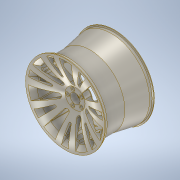
# Autodesk Inventor part: RIM
Saved by Autodesk Inventor 2020.2 (Build 242310000, 310)
## iProperties
RuleStatus: InUse
AfterAnyParamChange0: DARule
Created: 2019-05-23
Part Number: RIM
Material: Titanium
Document SubType Name: Modeling
Designer: Autodesk Developer Network
Density: 4.51 g/cm^3
Appearance: Titanium
Mass: 15996.9 g
Surface Area: 6136.53 cm^2
Volume: 3546.98 cm^3
Author: Autodesk Developer Network
Autodesk Inventor part; units mm, degrees
ref_plane "YZ Plane" through (0, 0, 0) normal (1, 0, 0) x (0, 1, 0)
ref_plane "XZ Plane" through (0, 0, 0) normal (0, 1, 0) x (-1, 0, 0)
sketch "Sketch1" plane through (0, 0, 0) normal (1, 0, 0) x (0, 1, 0)
  line L0 (203.2, 50.8) -> (203.2, 47.625)
  line L1 (203.2, 47.625) -> (196.85, 45.3138)
  line L2 (196.85, 45.3138) -> (196.85, 32.6138)
  line L3 (196.85, 32.6138) -> (177.8, 19.2748)
  line L4 (177.8, 19.2748) -> (177.8, -76.9759)
  line L5 (177.8, -76.9759) -> (196.85, -185.0138)
  line L6 (196.85, -185.0138) -> (196.85, -197.7138)
  line L7 (196.85, -197.7138) -> (203.2, -200.025)
  line L8 (203.2, -200.025) -> (203.2, -203.2)
  line L9 (203.2, -203.2) -> (190.5, -198.5776)
  line L10 (190.5, -198.5776) -> (190.5, -185.8776)
  line L11 (190.5, -185.8776) -> (158.75, -67.385)
  line L12 (158.75, -67.385) -> (158.75, 20.9537)
  line L13 (158.75, 20.9537) -> (165.1, 25.4)
  line L14 (165.1, 25.4) -> (154.94, 35.56)
  arc A0 (203.2, 50.8) -> (50.8, 0) centre (244.775, -327.9249) ccw
  arc A1 (154.94, 35.56) -> (50.8, -38.1) centre (319.7795, -307.9352) ccw
  line L15 (50.8, -38.1) -> (0, -38.1)
  line L16 (50.8, 0) -> (0, 0)
  line L17 (0, 0) -> (0, -38.1)
  dimension "w" = 254
  dimension "RimDia" = 203.2
  dimension "d2" = 381
  dimension "d3" = 381
  dimension "d5" = 6.35
  dimension "d6" = 110
  dimension "d7" = 3.175
  dimension "d8" = 3.175
  dimension "d9" = 110
  dimension "d10" = 19.05
  dimension "d11" = 125
  dimension "d14" = 12.7
  dimension "d15" = 50.8
  dimension "d16" = 38.1
  dimension "Width_angle2" = 170
  dimension "d18" = 12.7
  dimension "d19" = 6.35
  dimension "d20" = 19.05
  dimension "Width_angle1" = 165
  dimension "d22" = 125
  dimension "d24" = 50.8
  dimension "d25" = 50.8
  dimension "d28" = 38.1
  dimension "d29" = 25.4
  dimension "d30" = 48.26
  dimension "d31" = 15.24
  dimension "d32" = 18.1862
  constraints: 36 end point, 6 point on line, 5 parallel, 4 point on circle, 2 centre point, 2 horizontal, 1 perpendicular, 1 vertical
  measures "w" distance of L8.end L0.start
  measures "RimDia" horizontal distance of point (0, 0) L0.start
  measures "d2" radius of A0
  measures "d3" radius of A1
  measures "d5" distance between parallel lines of L0 L2
  measures "d6" angle of L2 L1
  measures "d7" distance of L0.start L0.end
  measures "d8" distance of L7.end L8.end
  measures "d9" angle of L6 L7
  measures "d10" distance between parallel lines of L4 L2
  measures "d11" angle of L4 L3
  measures "d14" distance of L1.end L2.end
  measures "d15" vertical distance of point (0, 0) L0.start
  measures "d16" distance of L16.end L15.end
  measures "Width_angle2" angle of L4 L5
  measures "d18" distance of L9.end L10.end
  measures "d19" distance between parallel lines of L10 L6
  measures "d20" distance between parallel lines of L12 L4
  measures "Width_angle1" angle of L11 L12
  measures "d22" angle of L12 L13
  measures "d24" distance of L15.start L15.end
  measures "d25" distance of L16.start L16.end
  measures "d28" horizontal distance of L0.start L13.end
  measures "d29" vertical distance of L13.end L0.start
  measures "d30" horizontal distance of L14.end L0.start
  measures "d31" vertical distance of L14.end L0.start
  measures "d32" vertical distance of L5.end L8.end
revolve "Revolution1" add sketch "Sketch1" angle 360 about axis through (0, 0, 0) along (0, 0, -1)
ref_plane "Work Plane1" through (0, 0, 127) normal (0, 0, 1) x (1, 0, 0)
sketch "Sketch2" plane through (0, 0, 127) normal (0, 0, 1) x (1, 0, 0)
  line L0 (0, 0) -> (0, 330.4538) construction
  line L1 (0, 0) -> (-140.0906, 300.4252) construction
  circle A0 centre (0, 0) radius 203.2 projected
  line L2 (-58.1057, 161.3035) -> (-36.8819, 93.9904)
  arc A1 (29.2479, 168.9369) -> (-29.2479, 168.9369) centre (0, 0) ccw
  arc A2 (-58.1057, 161.3035) -> (-86.2161, 148.1955) centre (0, 0) ccw
  line L3 (-29.2479, 168.9369) -> (-12.5071, 73.9947)
  line L4 (29.2479, 168.9369) -> (12.5071, 73.9947)
  arc A3 (-12.5071, 73.9947) -> (12.5071, 73.9947) centre (0, 76.2) ccw
  line L5 (-48.2936, 88.669) -> (-86.2161, 148.1955)
  arc A4 (-48.2936, 88.669) -> (-36.8819, 93.9904) centre (-42.938, 92.0809) ccw
  point P0 (0, 122.9635)
  dimension "d35" = 25
  dimension "Gap" = 31.75
  dimension "d43" = 31.75
  dimension "d79" = 20
  dimension "d80" = 12.7
  dimension "d81" = 76.2
  dimension "d97" = 6.35
  dimension "d98" = 101.6
  dimension "d99" = 15
  constraints: 12 end point, 8 point on circle, 4 centre point, 4 tangent, 3 point on line, 1 coincident, 1 horizontal alignment, 1 symmetric about line, 1 vertical, 1 vertical alignment
  measures "d35" angle of L0 L1
  measures "Gap" radial gap between concentric circles of A0 A1
  measures "d43" radial gap between concentric circles of A0 A2
  measures "d79" angle of L4 L3
  measures "d80" radius of A3
  measures "d81" distance of L0.start A3.centre
  measures "d97" radius of A4
  measures "d98" distance of A1.centre A4.centre
  measures "d99" angle of L5 L2
extrude "Extrusion1" cut sketch "Sketch2" against normal up to next contours L4 A3 L3 A1
chamfer "Chamfer1" distance 20.32 angle 45 2 edges at (14.6779, 170.8206, 45.9527) (-14.6779, 170.8206, 45.9527)
sketch "Sketch8" plane through (0, 0, 127) normal (0, 0, 1) x (1, 0, 0)
  line L0 (0, 0) -> (-85.876, 184.1617)
  line L1 (0, 0) -> (0, 203.2)
  circle A0 centre (0, 0) radius 203.2 projected
  line L2 (-70.5499, 121.2439) -> (-49.0809, 75.2035)
  line L3 (-26.0607, 85.938) -> (-47.5297, 131.9784)
  arc A1 (-49.0809, 75.2035) -> (-26.0607, 85.938) centre (-37.5708, 80.5708) ccw
  arc A2 (-47.5297, 131.9784) -> (-70.5499, 121.2439) centre (-59.0398, 126.6112) ccw
  dimension "d109" = 25
  dimension "d110" = 12.7
  dimension "d111" = 203.2
  dimension "d112" = 12.7
  dimension "Slot_Width" = 50.8
  dimension "Slot_Gap" = 63.5
  constraints: 8 end point, 4 point on circle, 4 tangent, 2 centre point, 2 point on line, 1 vertical, 1 vertical alignment, 1 other
  measures "d109" angle of L0 L1
  measures "d110" radius of A1
  measures "d111" distance of L0.start L0.end
  measures "d112" radius of A2
  measures "Slot_Width" distance of A1.centre A2.centre
  measures "Slot_Gap" distance of L0.end A2.centre
extrude "Extrusion7" [suppressed]
pattern_circular "Circular Pattern1" count 7 over 360 about axis through (0, 0, -28.8505) along (0, 0, -1) of "Extrusion1", "Chamfer1"
extrude "Extrusion6" cut sketch "Sketch2" against normal blind 228.6 contours L2 A4 L5 A2
chamfer "Chamfer4" distance 20.32 angle 45 1 edges at (-72.4579, 155.3865, 45.9527)
sketch "Sketch9" plane through (0, 0, 127) normal (0, 0, 1) x (1, 0, 0)
  line L0 (0, 0) -> (0, 203.2)
  circle A0 centre (0, 0) radius 203.2 projected
  line L1 (-12.7, 76.2) -> (-12.7, 139.7)
  line L2 (12.7, 76.2) -> (12.7, 139.7)
  arc A1 (12.7, 139.7) -> (-12.7, 139.7) centre (0, 139.7) ccw
  arc A2 (-12.7, 76.2) -> (12.7, 76.2) centre (0, 76.2) ccw
  dimension "d118" = 12.7
  dimension "Slot_Height" = 76.2
  dimension "d121" = 63.5
  constraints: 6 end point, 4 point on circle, 3 tangent, 3 vertical, 2 centre point, 1 equal radius, 1 point on line, 1 vertical alignment, 1 other
  measures "d118" radius of A1
  measures "Slot_Height" distance of A2.centre L0.start
  measures "d121" distance of A2.centre A1.centre
extrude "Extrusion8" [suppressed]
pattern_circular "Circular Pattern4" count 7 over 360 about axis through (0, 0, -327.9249) along (0, 0, -1) of "Extrusion6", "Chamfer4"
sketch "Sketch3" plane through (0, 0, 0) normal (0, 0, 1) x (1, 0, 0)
  circle A0 centre (-38.1, 0) radius 7.62
  point P0 (0, 0)
  dimension "d56" = 15.24
  dimension "d58" = 38.1
  dimension "d59" = 0
  constraints: 1 centre point
  measures "d56" diameter of A0
  measures "d58" distance of point (0, 0) A0.centre
  measures "d59" vertical distance of point (0, 0) A0.centre
extrude "Extrusion2" cut sketch "Sketch3" against normal blind 12.7
sketch "Sketch4" plane through (-38.1, 0, -12.7) normal (0, 0, 1) x (1, 0, 0)
  circle A0 centre (0, 0) radius 4.445
  circle A1 centre (0, 0) radius 7.62 projected
  point P0 (38.1, 0)
  dimension "d62" = 8.89
  constraints: 1 centre point, 1 concentric
  measures "d62" diameter of A0
extrude "Extrusion3" cut sketch "Sketch4" against normal up to next contours A0
chamfer "Chamfer2" distance 2.54 angle 45 1 edges at (-42.545, 0, -12.7)
pattern_circular "Circular Pattern2" count 5 over 360 about axis through (0, 0, -28.8505) along (0, 0, -1) of "Extrusion3", "Chamfer2", "Extrusion2"
sketch "Sketch5" plane through (0, 0, 0) normal (0, 0, 1) x (1, 0, 0)
  circle A0 centre (0, 0) radius 25.4
  dimension "d71" = 50.8
  constraints: 1 centre point, 1 coincident
  measures "d71" diameter of A0
extrude "Extrusion4" cut sketch "Sketch5" against normal up to next
fillet "Fillet3" radius 2.54 5 edges at (-14.1283, -43.4823, 0) (-45.72, 0, 0) (-14.1283, 43.4823, 0) (36.9883, 26.8735, 0) (36.9883, -26.8735, 0)
chamfer "Chamfer3" distance 5.08 angle 45 1 edges at (-25.4, 0, -38.1)
equation "\"Diameter\" = 406.4"
equation "\"Width\" = 254"
body "Solid1"
